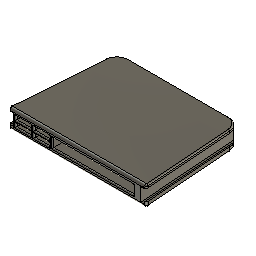
ID.3 Separator Badge (Autodesk Fusion 360 design; units mm, degrees)
part number: 2026-04-10-16-56-54-716
Autodesk Fusion 360 part; units mm, degrees
note: some values were not read from the file. Set by a fixed rule: which sketch regions a step uses.
sketch "Sketch1" plane through (0, 0, 0) normal (0, 0, 1) x (1, 0, 0)
  line L0 (0, 0) -> (0.0278, 83.3)
  line L1 (0.0278, 83.3) -> (40.7389, 83.2864)
  line L2 (50.7086, 74.0194) -> (56.15, -0.0187)
  line L3 (56.15, -0.0187) -> (0, 0)
  line L4 (-50.6592, 74.0532) -> (-56.15, 0.0187)
  line L5 (0, 0) -> (0.0278, 83.3)
  line L6 (0.0278, 83.3) -> (-40.6833, 83.3136)
  line L7 (-56.15, 0.0187) -> (0, 0)
  arc A0 (50.7086, 74.0194) -> (40.7389, 83.2864) centre (40.7355, 73.2864) ccw
  arc A1 (-40.6833, 83.3136) -> (-50.6592, 74.0532) centre (-40.6866, 73.3136) ccw
  point P0 (50.0278, 83.2833)
  dimension "d4" = 56.15
  dimension "d5" = 50
  dimension "d6" = 83.3
  dimension "d9" = 10
  dimension "d10" = 10
  constraint coincident L0.start L3.end
  constraint perpendicular L0 L1
  constraint perpendicular L0 L3
  constraint symmetric L3.end L0 L5.start
  constraint symmetric L1.start L0 L5.end
  constraint symmetric L0 L2.end L4.end
  constraint symmetric L0 L3.end L5.start
  constraint coincident P0 L1
  constraint coincident P0 L2
  constraint tangent L1 A0
  constraint tangent L2 A0
  constraint tangent L4 A1
  constraint tangent L6 A1
  measures "d4" horizontal distance of L2.end L0.start
  measures "d5" horizontal distance of L0.end P0
  measures "d6" vertical distance of L0.start L0.end
  measures "d9" radius of A0
  measures "d10" radius of A1
extrude "Extrude1" add sketch "Sketch1" along normal blind 15.7 makes body 1
sketch "Sketch2" plane through (55.847, 4.1044, 0) normal (0.99731, 0.073296, 0) x (-0.073296, 0.99731, 0)
  line L0 (-4.1343, 0) -> (70.1035, 0)
  line L1 (70.1035, 0) -> (70.1035, 15.7)
  line L2 (70.1035, 15.7) -> (-4.1343, 15.7)
  line L3 (-4.1343, 15.7) -> (-4.1343, 0)
  line L4 (-4.1343, 13.2) -> (85.8724, 13.2)
  line L5 (85.8724, 13.2) -> (85.8724, 3.7)
  line L6 (85.8724, 3.7) -> (-4.1343, 3.7)
  line L7 (-4.1343, 3.7) -> (-4.1343, 13.2)
  dimension "d13" = 2.5
  dimension "d14" = 3.7
  constraint horizontal L4
  constraint vertical L5
  constraint horizontal L6
  constraint vertical L7
  constraint coincident L3 L4.start
  measures "d13" distance of L2 L4
  measures "d14" distance of L0 L6
sketch "Sketch4" plane through (-55.8442, 4.1417, 0) normal (-0.997261, 0.073962, 0) x (-0.073962, -0.997261, 0)
  line L0 (-70.1035, 0) -> (4.1343, 0)
  line L1 (4.1343, 0) -> (4.1343, 15.7)
  line L2 (4.1343, 15.7) -> (-70.1035, 15.7)
  line L3 (-70.1035, 15.7) -> (-70.1035, 0)
  line L4 (4.1343, 13.2) -> (-93, 13.2)
  line L5 (-93, 13.2) -> (-93, 3.7)
  line L6 (-93, 3.7) -> (4.1343, 3.7)
  line L7 (4.1343, 3.7) -> (4.1343, 13.2)
  dimension "d17" = 2.5
  dimension "d18" = 3.7
  constraint horizontal L4
  constraint vertical L5
  constraint horizontal L6
  constraint vertical L7
  constraint coincident L1 L4.start
  measures "d17" distance of L2 L4
  measures "d18" distance of L0 L6
extrude "Extrude2" cut sketch "Sketch4" against normal blind 4 contours L3 L4 L5 L6 | L1 L3 L4 L6 L7 bodies 1
extrude "Extrude3" cut sketch "Sketch2" against normal blind 4 contours L1 L3 L4 L6 L7 | L1 L4 L5 L6 bodies 1
sketch "Sketch8" plane through (0, 0, 3.7) normal (0, 0, 1) x (-1, 0, 0)
  line L0 (-52.1391, 0.0174) -> (-56.15, 0.0187)
  line L1 (-56.15, 0.0187) -> (-50.7086, -74.0194)
  line L2 (-46.133, -81.7047) -> (-52.1391, 0.0174)
  line L3 (-52.1391, 0.0174) -> (-54.9543, 0.0183)
  line L4 (-48.933, -81.9105) -> (-46.133, -81.7047)
  line L5 (-46.133, -81.7047) -> (-52.1391, 0.0174)
  line L6 (-48.933, -81.9105) -> (-54.9543, 0.0183)
  line L7 (0, -88) -> (0, 10)
  line L8 (48.933, -81.9105) -> (54.9543, 0.0183)
  line L9 (48.933, -81.9105) -> (46.133, -81.7047)
  line L10 (46.133, -81.7047) -> (52.1391, 0.0174)
  line L11 (52.1391, 0.0174) -> (54.9543, 0.0183)
  arc A0 (-50.7086, -74.0194) -> (-46.133, -81.7047) centre (-40.7355, -73.2864) ccw
  dimension "d27" = 2.8
  constraint coincident L0.start L2.end
  constraint coincident L0 L3.end
  constraint coincident L2.start L4.end
  constraint vertical L7
  constraint parallel L5 L6
  constraint symmetric L0.start L7 L10.end
  constraint symmetric L3.end L7 L8.end
  constraint symmetric L4.start L7 L8.start
  constraint symmetric L2.start L7 L9.end
  measures "d27" horizontal distance of L4.start L2.start
extrude "Extrude4" cut sketch "Sketch8" against normal blind 1.5 contours L0 L2 L3 L5 L6 A0 | L8 L9 L10 L11 bodies 1
fillet "Fillet1" radius 2 6 edges at (0, 0, 0) (0, 0, 15.7) (56.15, -0.0187, 14.45) (56.15, -0.0187, 1.85) (-56.15, 0.0187, 1.85) (-56.15, 0.0187, 14.45) on bodies 1
fillet "Fillet2" radius 1 9 edges at (55.4113, 0.5673, 15.1142) (55.9962, 2.055, 15.7) (53.3504, 38.074, 15.7) (47.5438, 80.6109, 15.7) (0.0278, 83.3, 15.7) (-47.4899, 80.6426, 15.7) (-53.325, 38.1096, 15.7) (-55.9948, 2.0924, 15.7) (-55.4109, 0.6043, 15.1142) on bodies 1
fillet "Fillet3" radius 1 9 edges at (-55.4109, 0.6043, 0.5858) (-55.9948, 2.0924, 0) (-53.325, 38.1096, 0) (-47.4899, 80.6426, 0) (0.0278, 83.3, 0) (47.5438, 80.6109, 0) (53.3504, 38.074, 0) (55.9962, 2.055, 0) (55.4113, 0.5673, 0.5858) on bodies 1
copy_body "CopyPasteBodies2" bodies 1 makes body 2
sketch "Sketch9" plane through (0, 0, 0) normal (-0.000334, -1, 0) x (1, -0.000334, 0)
  line L0 (53.9969, 13.2) -> (53.9969, 13.7)
  line L1 (53.9969, 13.7) -> (-53.9969, 13.7)
  line L2 (-53.9969, 13.7) -> (-53.9969, 13.2)
  line L3 (-53.9969, 13.2) -> (-52.1391, 13.2)
  line L4 (-52.1391, 13.2) -> (-52.1391, 3.7)
  line L5 (-52.1391, 3.7) -> (-52.1366, 3.7)
  line L6 (-52.1366, 3.7) -> (-52.1366, 2.2)
  line L7 (-52.1366, 2.2) -> (-53.9969, 2.2)
  line L8 (-53.9969, 2.2) -> (-53.9969, 2)
  line L9 (-53.9969, 2) -> (53.9969, 2)
  line L10 (53.9969, 2) -> (53.9969, 2.2)
  line L11 (53.9969, 2.2) -> (52.1391, 2.2)
  line L12 (52.1391, 2.2) -> (52.1391, 13.2)
  line L13 (52.1391, 13.2) -> (53.9969, 13.2)
  line L14 (45.9005, 11.35) -> (-20.0995, 11.35)
  line L15 (-20.0995, 11.35) -> (-20.0995, 4.35)
  line L16 (-20.0995, 4.35) -> (45.9005, 4.35)
  line L17 (45.9005, 4.35) -> (45.9005, 11.35)
  line L18 (-50.1391, 11.7) -> (-38.1391, 11.7)
  line L19 (-38.1391, 11.7) -> (-38.1391, 9.05)
  line L20 (-38.1391, 9.05) -> (-50.1391, 9.05)
  line L21 (-50.1391, 9.05) -> (-50.1391, 11.7)
  line L22 (-23.1391, 9.05) -> (-35.1391, 9.05)
  line L23 (-35.1391, 9.05) -> (-35.1391, 11.7)
  line L24 (-35.1391, 11.7) -> (-23.1391, 11.7)
  line L25 (-23.1391, 11.7) -> (-23.1391, 9.05)
  line L26 (-23.1391, 4.05) -> (-35.1391, 4.05)
  line L27 (-35.1391, 4.05) -> (-35.1391, 6.7)
  line L28 (-35.1391, 6.7) -> (-23.1391, 6.7)
  line L29 (-23.1391, 6.7) -> (-23.1391, 4.05)
  line L30 (-50.1391, 4.05) -> (-50.1391, 6.7)
  line L31 (-50.1391, 6.7) -> (-38.1391, 6.7)
  line L32 (-38.1391, 6.7) -> (-38.1391, 4.05)
  line L33 (-38.1391, 4.05) -> (-50.1391, 4.05)
  dimension "d36" = 66
  dimension "d37" = 7
  dimension "d40" = 2.35
  dimension "d45" = 12
  dimension "d46" = 2.65
  dimension "d47" = 2
  dimension "d48" = 2
  dimension "d49" = 12
  dimension "d50" = 2.65
  dimension "d51" = 12
  dimension "d52" = 2.65
  dimension "d53" = 12
  dimension "d54" = 2.65
  constraint horizontal L14
  constraint vertical L15
  constraint horizontal L16
  constraint vertical L17
  constraint horizontal L18
  constraint vertical L19
  constraint horizontal L20
  constraint vertical L21
  constraint horizontal L24
  constraint vertical L25
  constraint horizontal L22
  constraint vertical L23
  constraint horizontal L28
  constraint vertical L29
  constraint horizontal L26
  constraint vertical L27
  constraint horizontal L31
  constraint vertical L32
  constraint horizontal L33
  constraint vertical L30
  measures "d36" distance of L14.start L14.end
  measures "d37" distance of L14.start L16.end
  measures "d40" distance of L1 L14
  measures "d45" distance of L18.start L18.end
  measures "d46" distance of L18.start L20.end
  measures "d47" distance of L1 L18
  measures "d48" distance of L4 L21
  measures "d49" distance of L23.end L24.end
  measures "d50" distance of L22.end L23.end
  measures "d51" distance of L27.end L28.end
  measures "d52" distance of L26.end L27.end
  measures "d53" distance of L30.end L31.end
  measures "d54" distance of L30.end L30.start
extrude "Extrude5" cut sketch "Sketch9" against normal blind 75 contours L14 L15 L16 L17 bodies 2
fillet "Fillet4" radius 1 4 edges at (12.9005, -0.0043, 11.35) (-20.0995, 0.0067, 7.85) (12.9005, -0.0043, 4.35) (45.9005, -0.0153, 7.85) on bodies 2
extrude "Extrude6" cut sketch "Sketch9" against normal blind 6 contours L18 L19 L20 L21 | L22 L23 L24 L25 | L26 L27 L28 L29 | L30 L31 L32 L33 bodies 2
fillet "Fillet5" radius 1 16 edges at (-29.1391, 0.0097, 11.7) (-35.1391, 0.0117, 10.375) (-29.1391, 0.0097, 9.05) (-23.1391, 0.0077, 10.375) (-23.1391, 0.0077, 5.375) (-29.1391, 0.0097, 6.7) (-29.1391, 0.0097, 4.05) (-35.1391, 0.0117, 5.375) (-44.1391, 0.0147, 6.7) (-38.1391, 0.0127, 5.375) (-44.1391, 0.0147, 4.05) (-50.1391, 0.0167, 5.375) (-50.1391, 0.0167, 10.375) (-44.1391, 0.0147, 11.7) (-44.1391, 0.0147, 9.05) (-38.1391, 0.0127, 10.375) on bodies 2
hidden bodies 1
equation "d4 = ( 112.3 / 2 ) * 1 mm"
equation "d5 = ( 100 / 2 ) * 1 mm"
named bodies: "SeparatorBody", "SeparatorBody_badge"
